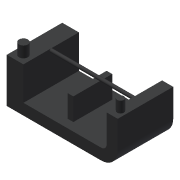
# Autodesk Inventor part: Interactice Exercise
Saved by Autodesk Inventor 2022 Beta2 (Build 260130000, 130) ContinuousBuild 0
## iProperties
Created: 2008-03-12
Part Number: Interactice Exercise
Document SubType Name: Modeling
Designer: jmacmillan
Density: 1 g/cm^3
Material: Generic
Appearance: Generic
Author: jmacmillan
Autodesk Inventor part; units mm, degrees
ref_plane "YZ Plane" through (0, 0, 0) normal (1, 0, 0) x (0, 1, 0)
ref_plane "XZ Plane" through (0, 0, 0) normal (0, 1, 0) x (-1, 0, 0)
ref_plane "XY Plane" through (0, 0, 0) normal (0, 0, 1) x (1, 0, 0)
sketch "Sketch1" plane through (0, 0, 0) normal (0, 1, 0) x (-1, 0, 0)
  line L0 (0, -140) -> (0, 140) projected
  line L1 (-350, 0) -> (350, 0) projected
  line L2 (-250, 100) -> (-250, -100)
  line L3 (-250, -100) -> (250, -100)
  line L4 (250, -100) -> (250, 100)
  line L5 (250, 100) -> (175, 100)
  line L6 (175, 100) -> (175, -50)
  line L7 (175, -50) -> (-200, -50)
  line L8 (-200, -50) -> (-200, 100)
  line L9 (-200, 100) -> (-250, 100)
  dimension "d0" = 200
  dimension "d1" = 50
  dimension "d2" = 50
  dimension "d3" = 500
  dimension "d4" = 75
  constraints: 16 end point, 7 parallel, 2 perpendicular, 2 other
  measures "d0" distance of L3.end L4.end
  measures "d1" distance between parallel lines of L3 L7
  measures "d2" distance of L8.end L2.start
  measures "d3" distance between parallel lines of L2 L4
  measures "d4" distance of L4.end L5.end
extrude "Extrusion1" add sketch "Sketch1" along normal mid plane 250 contours L3 L2 L1 L8 L7 L0 | L0 L7 L6 L1 L4 L3 | L2 L9 L8 L1 | L1 L6 L5 L4
fillet "Fillet1" radius 75 1 edges at (250, 0, -100)
fillet "Fillet1" radius 25 1 edges at (200, 0, -50)
sketch "Sketch2" plane through (-250, 125, 100) normal (0, 0, 1) x (1, 0, 0)
  line L0 (0, -250) -> (0, 0) projected
  line L1 (0, -250) -> (75, -250) projected
  line L2 (75, -250) -> (75, 0) projected
  circle A0 centre (37.5, -212.5) radius 37.5 construction
  circle A1 centre (37.5, -212.5) radius 20
  dimension "d9" = 40
  constraints: 3 tangent, 2 centre point, 1 coincident
  measures "d9" diameter of A1
extrude "Extrusion2" add sketch "Sketch2" along normal blind 50
sketch "Sketch3" plane through (200, 125, 100) normal (0, 0, 1) x (1, 0, 0)
  line L0 (0, -250) -> (50, -250) projected
  circle A0 centre (-412.5, -212.5) radius 20 projected
  circle A1 centre (25, -212.5) radius 15
  point P0 (25, -250)
  dimension "d12" = 30
  constraints: 1 centre point, 1 horizontal alignment, 1 midpoint, 1 vertical alignment
  measures "d12" diameter of A1
extrude "Extrusion3" add sketch "Sketch3" along normal up to surface (50 mm away) contours A1
sketch "Sketch4" plane through (0, 0, 0) normal (0, 1, 0) x (-1, 0, 0)
  line L0 (-175, -50) -> (175, -50) projected
  line L1 (-12.5, -50) -> (12.5, -50)
  line L2 (12.5, -50) -> (12.5, 50)
  line L3 (12.5, 50) -> (-12.5, 50)
  line L4 (-12.5, 50) -> (-12.5, -50)
  line L5 (0, -150) -> (0, 200) projected
  dimension "d15" = 25
  dimension "d16" = 100
  constraints: 8 end point, 2 parallel, 1 horizontal, 1 perpendicular, 1 point on line, 1 other
  measures "d15" distance of L2.end L3.end
  measures "d16" distance of L1.end L2.end
extrude "Extrusion4" add sketch "Sketch4" along normal mid plane 175
sketch "Sketch5" plane through (-175, -125, 100) normal (1, 0, 0) x (0, 0, -1)
  circle A0 centre (7.5, 125) radius 7.5
  line L0 (0, 250) -> (0, 0) projected
  point P0 (0, 125)
  dimension "d19" = 15
  constraints: 1 centre point, 1 horizontal alignment, 1 midpoint, 1 tangent
  measures "d19" diameter of A0
extrude "Extrusion5" add sketch "Sketch5" along normal up to next
body "Solid1"
